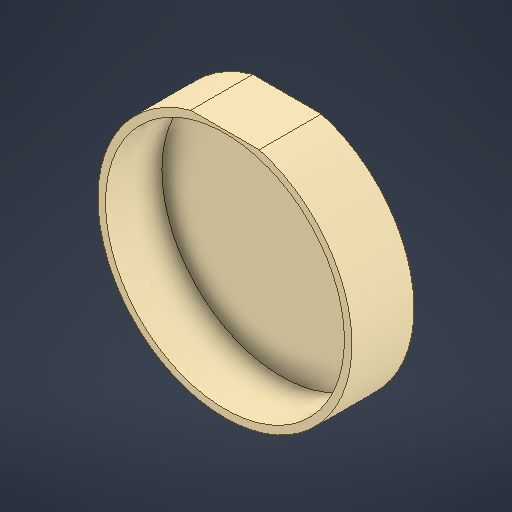
# Autodesk Inventor part: Miska
Saved by Autodesk Inventor 2026.2 (Build 302298000, 298)
## iProperties
Created: 2025-09-11
Part Number: Miska
Material: Všeobecné
Document SubType Name: Modeling
Designer: cerna
Density: 1 g/cm^3
Appearance: Béžová
Author: cerna
Autodesk Inventor part; units mm, degrees
ref_plane "YZ Plane" through (0, 0, 0) normal (1, 0, 0) x (0, 1, 0)
ref_plane "XZ Plane" through (0, 0, 0) normal (0, 1, 0) x (-1, 0, 0)
ref_plane "XY Plane" through (0, 0, 0) normal (0, 0, 1) x (1, 0, 0)
sketch "Náčrt1" plane through (0, 0, 0) normal (0, 0, 1) x (1, 0, 0)
  line L0 (0, 95.014) -> (0, -94.5857) projected
  line L1 (-94.5, 0) -> (94.5, 0) projected
  circle A0 centre (0, 0) radius 63.5
  arc A1 (-53.5, 41.1582) -> (53.5, 41.1582) centre (0, 0) ccw
  line L2 (-18.2003, 65) -> (18.2003, 65)
  arc A2 (53.8673, 40.6764) -> (18.2003, 65) centre (0, 0) ccw
  arc A3 (-18.2003, 65) -> (-53.5, 41.1582) centre (0, 0) ccw
  point P0 (53.5, 41.1582)
  dimension "d0" = 127
  dimension "d1" = 135
  dimension "d2" = 107
  dimension "d8" = 65
  constraints: 6 point on circle, 4 centre point, 3 coincident, 2 end point, 1 horizontal
  measures "d0" diameter of A0
  measures "d1" diameter of A1
  measures "d2" distance of A1.start A1.end
  measures "d8" distance from line of L2 A2.centre
extrude "Vysunutí1" add sketch "Náčrt1" along normal blind 3
sketch "Náčrt2" plane through (0, 0, 3) normal (0, 0, 1) x (1, 0, 0)
  circle A0 centre (0, 0) radius 63.5
  arc A1 (-18.2003, 65) -> (18.2003, 65) centre (0, 0) ccw projected
  line L0 (18.2003, 65) -> (-18.2003, 65) projected
  line L1 (-18.2003, 65) -> (18.2003, 65)
  line L2 (18.2003, 65) -> (-18.2003, 65)
  circle A2 centre (0, 0) radius 67.5
  circle A3 centre (0, 0) radius 63.5
  point P0 (53.5, 72.3723)
  point P1 (-53.5, 72.3723)
  dimension "d5" = 127
  constraints: 4 end point, 3 centre point, 3 coincident, 2 collinear, 2 concentric
  measures "d5" diameter of A0
extrude "Vysunutí2" add sketch "Náčrt2" along normal blind 30 contours L0 A1
